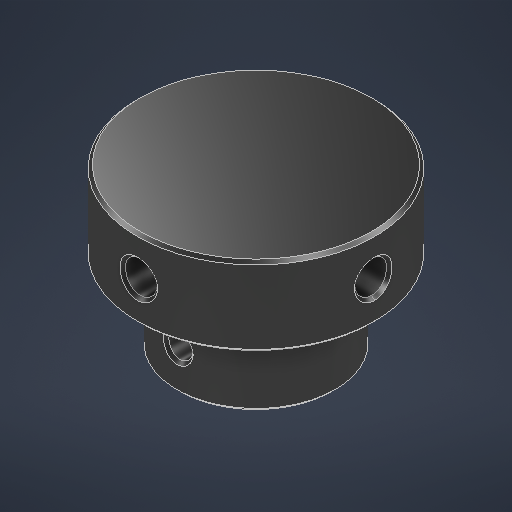
# Autodesk Inventor part: Part6
Saved by Autodesk Inventor 2026.2 (Build 302298010, 298A)
## iProperties
Created: 2026-03-22
Part Number: Part6
Material: Generic
Document SubType Name: Modeling
Designer: Mlinč
Density: 1 g/cm^3
Appearance: Default
Author: Mlinč
Autodesk Inventor part; units mm, degrees
ref_plane "YZ Plane" through (0, 0, 0) normal (1, 0, 0) x (0, 1, 0)
ref_plane "XZ Plane" through (0, 0, 0) normal (0, 1, 0) x (-1, 0, 0)
sketch "Sketch1" plane through (0, 0, 0) normal (0, 0, 1) x (1, 0, 0)
  line L0 (0, 0) -> (-20, 0)
  line L1 (-20, 0) -> (-20, 20)
  line L2 (-20, 20) -> (-30, 20)
  line L3 (-30, 20) -> (-30, 40)
  line L4 (-30, 40) -> (0, 40)
  line L5 (0, 40) -> (0, 0)
  dimension "d0" = 40
  dimension "d1" = 20
  dimension "d2" = 60
  dimension "d3" = 40
  constraints: 12 end point, 5 perpendicular, 1 horizontal
  measures "d0" distance of L4.end L0.start
  measures "d1" distance of L2.end L3.end
  measures "d2" diameter of L3 L5
  measures "d3" diameter of L1 L5
revolve "Revolution1" add sketch "Sketch1" angle 360 about axis through (0, 40, 0) along (0, -1, 0)
sketch "Sketch2" plane through (0, 0, 0) normal (0, -1, 0) x (1, 0, 0)
  circle A0 centre (0, 0) radius 8.5
  dimension "d5" = 17
  constraints: 1 centre point, 1 coincident
  measures "d5" diameter of A0
extrude "Extrusion1" cut sketch "Sketch2" against normal blind 20
ref_plane "Work Plane1" through (0, 10, 20) normal (0, 0, 1) x (1, 0, 0)
sketch "Sketch3" plane through (0, 10, 20) normal (0, 0, 1) x (1, 0, 0)
  circle A0 centre (0, 0) radius 3
  line L0 (-20, -10) -> (20, -10) projected
  point P0 (0, -10)
  dimension "d8" = 6
  dimension "d9" = 10
  constraints: 1 centre point, 1 vertical alignment
  measures "d8" diameter of A0
  measures "d9" distance from line of L0 A0.centre
extrude "Extrusion2" cut sketch "Sketch3" against normal through all
ref_plane "Work Plane2" through (0, 30, 30) normal (0, 0, 1) x (1, 0, 0)
sketch "Sketch4" plane through (0, 30, 30) normal (0, 0, 1) x (1, 0, 0)
  circle A0 centre (0, 0) radius 4
  line L0 (-30, 10) -> (30, 10) projected
  point P0 (0, -30)
  dimension "d12" = 8
  dimension "d13" = 10
  constraints: 1 centre point, 1 vertical alignment
  measures "d12" diameter of A0
  measures "d13" distance from line of L0 A0.centre
extrude "Extrusion3" cut sketch "Sketch4" against normal blind 10
pattern_circular "Circular Pattern1" count 4 over 360 about axis through (0, 30, 0) along (0, -1, 0) of "Extrusion3"
chamfer "Chamfer2" distance 0.75 angle 45 23 edges at (20, 0, 0) (-8.5, 0, 0) (20, 20, 0) (30, 20, 0) (30, 40, 0) (-29.7321, 30, -4) (-29.8448, 27.4095, 3.0478) (-29.845, 32.5926, 3.0461) (-3.0573, 32.5794, -29.8438) (-3.0552, 27.4182, -29.844) (3.9999, 30.0316, -29.7322) (29.845, 32.5926, -3.0461) (29.7321, 30, 4) (29.8448, 27.4095, -3.0478) (3.0573, 32.5794, 29.8438) (3.0552, 27.4182, 29.844) (-3.9999, 30.0316, 29.7322) (-2.9999, 10.029, -19.7737) (2.244, 11.9911, 19.8737) (-3, 10.0067, 19.7737) (2.2804, 8.0507, 19.8696) (-3, 10.0046, 7.953) (-3, 10.0046, -7.953)
body "Solid1"
